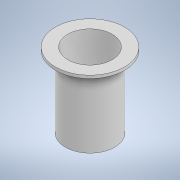
# Autodesk Inventor part: 62. Втулка рычага управления
Saved by Autodesk Inventor 2021 (Build 250183000, 183)
## iProperties
Created: 2021-03-10
Part Number: 62. Втулка рычага управления
Material: Типовые
Document SubType Name: Modeling
Designer: Данил
Density: 1 g/cm^3
Appearance: По умолчанию
Author: Данил
Autodesk Inventor part; units mm, degrees
ref_plane "YZ Plane" through (0, 0, 0) normal (1, 0, 0) x (0, 1, 0)
ref_plane "XZ Plane" through (0, 0, 0) normal (0, 1, 0) x (-1, 0, 0)
ref_plane "XY Plane" through (0, 0, 0) normal (0, 0, 1) x (1, 0, 0)
sketch "Эскиз1" plane through (0, 0, 0) normal (0, 0, 1) x (1, 0, 0)
  line L0 (0, 15.1) -> (0, -15.1)
  line L1 (10, -15.1) -> (10, 13.9)
  line L2 (10, 13.9) -> (14, 13.9)
  line L3 (14, 13.9) -> (14, 15.1)
  line L4 (14, 15.1) -> (9, 15.1)
  line L5 (9, 15.1) -> (9, -15.1)
  line L6 (9, -15.1) -> (10, -15.1)
  point P0 (0, 0)
  point P1 (0, 0)
  dimension "d0" = 30.2
  dimension "d1" = 18
  dimension "d2" = 20
  dimension "d3" = 29
  dimension "d4" = 28
  constraints: 14 end point, 5 perpendicular, 2 horizontal alignment, 2 vertical, 1 coincident, 1 midpoint
  measures "d0" distance of L0.start L0.end
  measures "d1" diameter of L5 L0
  measures "d2" diameter of L1 L0
  measures "d3" distance between parallel lines of L6 L2
  measures "d4" diameter of L3 L0
revolve "Вращение1" add sketch "Эскиз1" angle 360 about axis through (0, 15.1, 0) along (0, -1, 0)
